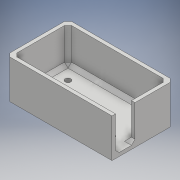
# Autodesk Inventor part: LiFeCase
Saved by Autodesk Inventor 2018 (Build 220112000, 112)
## iProperties
Created: 2018-08-30
Part Number: LiFeCase
Material: 一般
Document SubType Name: Modeling
Designer: shun2
Density: 1 g/cm^3
Appearance: 既定
Author: shun2
Autodesk Inventor part; units mm, degrees
ref_plane "YZ Plane" through (0, 0, 0) normal (1, 0, 0) x (0, 1, 0)
ref_plane "XZ Plane" through (0, 0, 0) normal (0, 1, 0) x (-1, 0, 0)
ref_plane "XY Plane" through (0, 0, 0) normal (0, 0, 1) x (1, 0, 0)
sketch "スケッチ1" plane through (0, 0, 0) normal (0, 0, 1) x (1, 0, 0)
  line L0 (0, 0) -> (60, 0)
  line L1 (60, 0) -> (60, 35)
  line L2 (60, 35) -> (0, 35)
  line L3 (0, 35) -> (0, 0)
  dimension "d0" = 60
  dimension "d1" = 35
  constraints: 8 end point, 2 parallel, 1 horizontal, 1 perpendicular
  measures "d0" distance of L2.end L1.end
  measures "d1" distance of L1.end L0.end
extrude "押し出し1" add sketch "スケッチ1" along normal blind 2
sketch "スケッチ2" plane through (0, 0, 2) normal (0, 0, 1) x (1, 0, 0)
  line L0 (60, 35) -> (0, 35) projected
  line L1 (2, 33) -> (2, 2)
  line L2 (0, 35) -> (0, 0) projected
  line L3 (58, 33) -> (58, 13.0563)
  line L4 (60, 0) -> (60, 35) projected
  line L5 (2, 33) -> (58, 33)
  line L6 (2, 2) -> (58, 2)
  line L7 (0, 0) -> (60, 0) projected
  line L8 (58, 13.0563) -> (60, 13.0563)
  line L9 (60, 2) -> (58, 2)
  line L10 (0, 35) -> (60, 35)
  line L11 (60, 0) -> (0, 0)
  line L12 (0, 0) -> (0, 35)
  line L13 (60, 13.0563) -> (58, 13.0563)
  line L14 (60, 2) -> (2, 2)
  line L15 (60, 35) -> (60, 13.0563)
  line L16 (60, 2) -> (60, 0)
  dimension "d4" = 2
  dimension "d5" = 2
  dimension "d6" = 2
  constraints: 26 end point, 5 perpendicular, 4 parallel, 3 horizontal, 1 collinear, 1 point on line, 1 vertical, 1 other
  measures "d4" distance between parallel lines of L1 L2
  measures "d5" distance between parallel lines of L4 L3
  measures "d6" distance between parallel lines of L5 L0
extrude "押し出し3" add sketch "スケッチ2" along normal blind 20 contours L4 L8 L3 L5 L1 L6 L9 L7 L2 L0
sketch "スケッチ3" plane through (0, 0, 2) normal (0, 0, 1) x (1, 0, 0)
  circle A0 centre (10, 25) radius 1.6
  line L0 (60, 35) -> (0, 35) projected
  line L1 (0, 35) -> (0, 0) projected
  circle A1 centre (50, 25) radius 1.6
  circle A2 centre (10, 10) radius 1.6
  circle A3 centre (50, 10) radius 1.6
  dimension "d12" = 3.2
  dimension "d13" = 10
  dimension "d14" = 10
  dimension "d15" = 3.2
  dimension "d16" = 3.2
  dimension "d17" = 3.2
  constraints: 4 centre point
  measures "d12" diameter of A0
  measures "d13" distance from line of L0 A0.centre
  measures "d14" distance from line of L1 A0.centre
  measures "d15" diameter of A1
  measures "d16" diameter of A2
  measures "d17" diameter of A3
extrude "押し出し4" cut sketch "スケッチ3" against normal blind 2
chamfer "面取り1" distance 2 angle 45 7 edges at (2, 17.5, 2) (30, 33, 2) (31, 2, 2) (2, 2, 12) (2, 33, 12) (60, 35, 11) (58, 23.0282, 2)
chamfer "面取り2" distance 2 angle 45 2 edges at (59, 13.0563, 2) (58, 33, 13)
chamfer "面取り3" distance 2 angle 45 2 edges at (0, 0, 11) (0, 35, 11)
